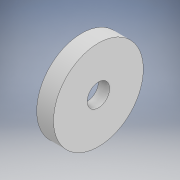
# Autodesk Inventor part: Rubber_Gromment_Cap_LM6015
Saved by Autodesk Inventor 2020.2 (Build 242310000, 310)
## iProperties
Created: 2020-04-20
Part Number: Rubber_Gromment_Cap_LM6015
Material: Generic
Document SubType Name: Modeling
Designer: rah75
Density: 1 g/cm^3
Appearance: Default
Author: rah75
Autodesk Inventor part; units mm, degrees
ref_plane "YZ Plane" through (0, 0, 0) normal (1, 0, 0) x (0, 1, 0)
ref_plane "XZ Plane" through (0, 0, 0) normal (0, 1, 0) x (-1, 0, 0)
ref_plane "XY Plane" through (0, 0, 0) normal (0, 0, 1) x (1, 0, 0)
sketch "Sketch1" plane through (0, 0, 0) normal (0, 0, 1) x (1, 0, 0)
  line L0 (-2, 2) -> (-2, 7)
  line L1 (-2, 7) -> (-3, 7)
  line L2 (-3, 7) -> (-3, 8)
  line L3 (-3, 8) -> (0, 8)
  line L4 (0, 8) -> (0, 2)
  line L5 (0, 2) -> (-2, 2)
  line L6 (0, 0) -> (-1.3687, 0) construction
  dimension "d0" = 14
  dimension "d1" = 1
  dimension "d2" = 1
  dimension "d3" = 2
  dimension "d4" = 4
  constraints: 14 end point, 5 perpendicular, 1 horizontal, 1 point on line, 1 vertical
  measures "d0" diameter of L1 L6
  measures "d1" distance of L0.end L1.end
  measures "d2" distance of L1.end L2.end
  measures "d3" distance of L4.end L0.start
  measures "d4" diameter of L5 L6
revolve "Revolution1" add sketch "Sketch1" angle 360 about axis through (0, 0, 0) along (-1, 0, 0)
body "Solid1"
